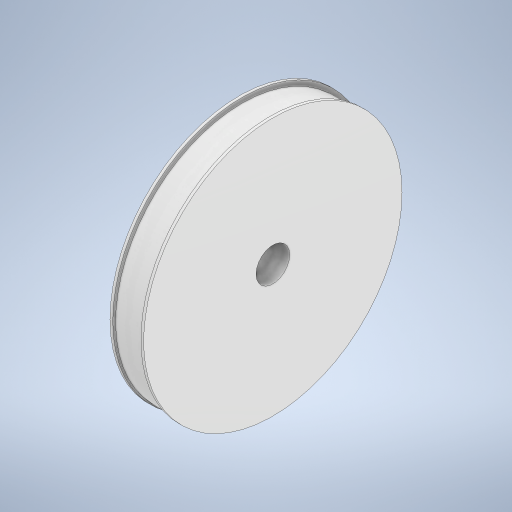
# Autodesk Inventor part: type3
Saved by Autodesk Inventor 2023 (Build 270158000, 158)
## iProperties
Created: 2022-04-24
Part Number: type3
Material: アセタール樹脂、白
Document SubType Name: Sheet Metal
Designer: yuta
Density: 1.425 g/cm^3
Sheet Metal Rule: Default_mm
Appearance: 滑らか - 白
Author: yuta
Autodesk Inventor part; units mm, degrees
ref_plane "YZ Plane" through (0, 0, 0) normal (1, 0, 0) x (0, 1, 0)
ref_plane "XZ Plane" through (0, 0, 0) normal (0, 1, 0) x (-1, 0, 0)
ref_plane "XY Plane" through (0, 0, 0) normal (0, 0, 1) x (1, 0, 0)
sketch "スケッチ1" plane through (0, 0, 0) normal (1, 0, 0) x (0, 1, 0)
  circle A0 centre (0, 0) radius 45
  dimension "d0" = 90
  constraints: 1 centre point, 1 coincident
  measures "d0" diameter of A0
extrude "押し出し1" add sketch "スケッチ1" along normal blind 10
sketch "スケッチ2" plane through (10, 0, 0) normal (1, 0, 0) x (0, 0, -1)
  circle A0 centre (0, 0) radius 46
  dimension "d3" = 92
  constraints: 1 centre point, 1 coincident
  measures "d3" diameter of A0
extrude "押し出し2" add sketch "スケッチ2" along normal blind 1
sketch "スケッチ3" plane through (0, 0, 0) normal (-1, 0, 0) x (0, 0, 1)
  circle A0 centre (0, 0.7888) radius 46
  point P0 (0, 0)
  dimension "d6" = 92
  constraints: 1 centre point
  measures "d6" diameter of A0
extrude "押し出し3" add sketch "スケッチ3" along normal blind 1
sketch "スケッチ4" plane through (-1, 0.7888, 0) normal (-1, 0, 0) x (0, 0, 1)
  point P0 (0, -0.7888)
sketch "スケッチ5" plane through (-1, 0.7888, 0) normal (-1, 0, 0) x (0, 0, 1)
  circle A0 centre (0, 0) radius 6
  circle A1 centre (0, 0) radius 46 projected
  point P0 (0, -0.7888)
  dimension "d9" = 12
  dimension "d10" = 40
  constraints: 1 centre point
  measures "d9" diameter of A0
  measures "d10" radial gap between concentric circles of A0 A1
extrude "押し出し4" cut sketch "スケッチ5" against normal blind 12 contours A0
equation "\"BendRadius\" = Thickness"
equation "\"BendReliefWidth\" = Thickness"
equation "\"BendReliefDepth\" = 0.5 * Thickness"
equation "\"CornerReliefSize\" = 4 * Thickness"
equation "\"MinimumRemnant\" = 2 * Thickness"
equation "\"TransitionRadius\" = BendRadius"
equation "\"JacobiRadiusSize\" = BendRadius"
equation "\"GapSize\" = Thickness"
equation "\"Thickness\" = 0.5"
